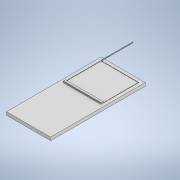
# Autodesk Inventor part: mousetrap
Saved by Autodesk Inventor 2021 (Build 250183000, 183)
## iProperties
Created: 2021-02-20
Part Number: mousetrap
Material: Generic
Document SubType Name: Modeling
Designer: bagal
Density: 1 g/cm^3
Appearance: Default
Author: bagal
Autodesk Inventor part; units mm, degrees
ref_plane "YZ Plane" through (0, 0, 0) normal (1, 0, 0) x (0, 1, 0)
ref_plane "XZ Plane" through (0, 0, 0) normal (0, 1, 0) x (-1, 0, 0)
ref_plane "XY Plane" through (0, 0, 0) normal (0, 0, 1) x (1, 0, 0)
sketch "Sketch1" plane through (0, 0, 0) normal (0, 1, 0) x (-1, 0, 0)
  line L0 (5.3777, 6.5934) -> (5.3777, -88.6566)
  line L1 (5.3777, -88.6566) -> (-39.0723, -88.6566)
  line L2 (-39.0723, -88.6566) -> (-39.0723, 6.5934)
  line L3 (-39.0723, 6.5934) -> (5.3777, 6.5934)
  point P0 (0, 0)
  dimension "d0" = 95.25
  dimension "d1" = 44.45
  constraints: 8 end point, 3 perpendicular, 1 vertical
  measures "d0" distance of L0.start L0.end
  measures "d1" distance of L0.end L1.end
extrude "Extrusion1" add sketch "Sketch1" along normal blind 3.175
sketch "Sketch2" plane through (0, 3.175, 0) normal (0, 1, 0) x (1, 0, 0)
  line L0 (39.0723, 88.6566) -> (-5.3777, 88.6566) projected
  line L1 (-5.3777, 88.6566) -> (-2.2027, 88.6566)
  line L2 (-2.2027, 88.6566) -> (-2.2027, 85.4816)
  line L3 (-2.2027, 85.4816) -> (-1.9487, 85.4816)
  line L4 (-1.9487, 85.4816) -> (-1.9487, 49.9216)
  line L5 (-1.9487, 49.9216) -> (-2.2027, 49.9216)
  line L6 (-2.2027, 49.9216) -> (-2.2027, 85.4816)
  point P0 (0, 0)
  dimension "d4" = 3.175
  dimension "d5" = 3.175
  dimension "d6" = 0.254
  dimension "d7" = 35.56
  dimension "d8" = 35.56
  constraints: 12 end point, 4 perpendicular, 1 horizontal, 1 point on line
  measures "d4" distance of L0.end L1.end
  measures "d5" distance of L1.end L2.end
  measures "d6" distance of L2.end L3.end
  measures "d7" distance of L3.end L4.end
  measures "d8" distance of L5.end L2.end
extrude "Extrusion2" add sketch "Sketch2" along normal blind 0.254
fillet "Fillet1" radius 0.127 2 edges at (-1.9487, 3.429, -67.7016) (-2.2027, 3.429, -67.7016)
sketch "Sketch3" plane through (0, 3.175, 0) normal (0, 1, 0) x (1, 0, 0)
  line L0 (39.0723, -6.5934) -> (39.0723, 88.6566) projected
  line L1 (39.0723, 88.6566) -> (35.9091, 88.6566)
  line L2 (39.0723, 88.6566) -> (-5.3777, 88.6566) projected
  line L3 (35.9091, 88.6566) -> (35.9091, 85.4816)
  line L4 (35.9091, 85.4816) -> (35.6551, 85.4816)
  line L5 (35.6551, 85.4816) -> (35.6551, 49.9216)
  line L6 (35.6551, 49.9216) -> (35.9091, 49.9216)
  line L7 (35.9091, 49.9216) -> (35.9091, 85.4816)
  point P0 (0, 0)
  dimension "d12" = 3.175
  dimension "d13" = 0.254
  dimension "d14" = 35.56
  dimension "d15" = 0.254
  dimension "d16" = 35.56
  constraints: 12 end point, 3 perpendicular, 1 horizontal, 1 point on line
  measures "d12" distance of L1.end L3.end
  measures "d13" distance of L3.end L4.end
  measures "d14" distance of L4.end L5.end
  measures "d15" distance of L5.end L6.end
  measures "d16" distance of L6.end L3.end
extrude "Extrusion3" add sketch "Sketch3" along normal blind 0.254
fillet "Fillet2" radius 0.127 2 edges at (35.9091, 3.429, -67.7016) (35.6551, 3.429, -67.7016)
sketch "Sketch4" plane through (0, 3.175, 0) normal (0, 1, 0) x (1, 0, 0)
  line L0 (-1.9487, 85.4816) -> (-1.9487, 49.9216) projected
  line L1 (35.6551, 49.9216) -> (35.6551, 85.4816) projected
  line L2 (-1.9487, 85.4816) -> (35.6551, 85.4816)
  line L3 (35.6551, 85.4816) -> (35.6551, 85.2276)
  line L4 (35.6551, 85.2276) -> (-1.9487, 85.2276)
  line L5 (-1.9487, 85.2276) -> (-1.9487, 85.4816)
  point P0 (0, 0)
  dimension "d20" = 0.254
  constraints: 8 end point, 2 perpendicular, 1 horizontal, 1 point on line
  measures "d20" distance of L1.end L3.end
extrude "Extrusion4" add sketch "Sketch4" along normal blind 0.254
fillet "Fillet3" radius 0.127 2 edges at (16.8532, 3.429, -85.2276) (16.8532, 3.429, -85.4816)
sketch "Sketch5" plane through (-2.2027, 3.175, -85.4816) normal (-1, 0, 0) x (0, 0, 1)
  point P0 (85.4816, -3.175)
sketch "Sketch6" plane through (0, 3.175, 0) normal (0, 1, 0) x (1, 0, 0)
  line L0 (-2.2027, 85.4816) -> (-1.9487, 85.4816) projected
  line L1 (-2.2027, 85.4816) -> (-2.4567, 85.4816)
  line L2 (35.6551, 85.4816) -> (-1.9487, 85.4816) projected
  line L3 (-1.9487, 85.4816) -> (-1.6947, 85.4816)
  line L4 (-1.6947, 85.4816) -> (-1.6947, 117.2316)
  line L5 (-2.2027, 85.4816) -> (-2.2027, 117.2316)
  line L6 (-2.2027, 117.2316) -> (-1.6947, 117.2316)
  point P0 (0, 0)
  dimension "d24" = 0.254
  dimension "d25" = 0.254
  dimension "d26" = 31.75
  constraints: 10 end point, 2 perpendicular, 1 horizontal, 1 parallel, 1 point on line
  measures "d24" distance of L0.start L1.end
  measures "d25" distance of L0.end L3.end
  measures "d26" distance of L3.end L4.end
extrude "Extrusion5" add sketch "Sketch6" along normal blind 0.508
fillet "Fillet4" radius 0.127 1 edges at (-1.9487, 3.683, -85.4816)
sketch "Sketch7" plane through (0, 3.683, 0) normal (0, 1, 0) x (1, 0, 0)
  line L0 (-2.2027, 117.2316) -> (-2.2027, 88.6566) projected
  line L1 (-2.2027, 117.2316) -> (-2.2027, 114.0566)
  line L2 (-2.2027, 114.0566) -> (-1.6947, 114.0566)
  line L3 (-1.6947, 85.6086) -> (-1.6947, 117.2316) projected
  line L4 (-2.2027, 114.0566) -> (-2.2027, 113.8026)
  line L5 (-2.2027, 113.8026) -> (-1.6947, 113.8026)
  line L6 (-1.6947, 113.8026) -> (-1.6947, 114.0566)
  point P0 (0, 0)
  dimension "d30" = 3.175
  dimension "d31" = 0.254
  constraints: 10 end point, 3 perpendicular, 3 point on line
  measures "d30" distance of L0.start L1.end
  measures "d31" distance of L1.end L4.end
extrude "Extrusion6" cut sketch "Sketch7" against normal blind 0.254
sketch "Sketch8" plane through (0, 3.683, 0) normal (0, 1, 0) x (1, 0, 0)
  line L0 (-1.6947, 113.8026) -> (-2.2027, 113.8026) projected
  line L1 (-2.2027, 113.8026) -> (-2.2027, 107.4526)
  line L2 (-2.2027, 117.2316) -> (-2.2027, 88.6566) projected
  line L3 (-2.2027, 107.4526) -> (-1.6947, 107.4526)
  line L4 (-1.6947, 88.6566) -> (-1.6947, 117.2316) projected
  line L5 (-2.2027, 107.4526) -> (-2.2027, 107.1986)
  line L6 (-2.2027, 107.1986) -> (-1.6947, 107.1986)
  line L7 (-1.6947, 107.4526) -> (-1.6947, 107.1986)
  line L8 (-2.2027, 107.4526) -> (-1.6947, 107.4526)
  line L9 (-1.6947, 107.1986) -> (-1.6947, 107.4526)
  line L10 (-2.2027, 107.4526) -> (-2.2027, 107.1986)
  line L11 (-2.2027, 107.1986) -> (-1.6947, 107.1986)
  point P0 (0, 0)
  dimension "d34" = 6.35
  dimension "d35" = 0.254
  constraints: 18 end point, 4 collinear, 4 point on line, 3 perpendicular
  measures "d34" distance of L0.end L1.end
  measures "d35" distance of L1.end L5.end
extrude "Extrusion7" cut sketch "Sketch8" against normal blind 0.254 contours L4 L6 L2 L3
sketch "Sketch9" plane through (0, 3.175, 0) normal (0, 1, 0) x (1, 0, 0)
  line L0 (-2.2027, 85.4816) -> (-2.2027, 49.9216) projected
  line L1 (35.9091, 49.9216) -> (35.6551, 49.9216) projected
  line L2 (-2.2027, 49.9216) -> (35.9091, 49.9216)
  line L3 (35.9091, 49.9216) -> (35.9091, 47.3816)
  line L4 (35.9091, 47.3816) -> (-2.2027, 47.3816)
  line L5 (-2.2027, 47.3816) -> (-2.2027, 49.9216)
  point P0 (0, 0)
  dimension "d38" = 2.54
  constraints: 8 end point, 3 perpendicular, 1 horizontal
  measures "d38" distance of L1.start L3.end
extrude "Extrusion8" add sketch "Sketch9" along normal blind 1.27
fillet "Fillet5" radius 0.254 2 edges at (16.8532, 4.445, -47.3816) (16.8532, 4.445, -49.9216)
body "Solid1"
